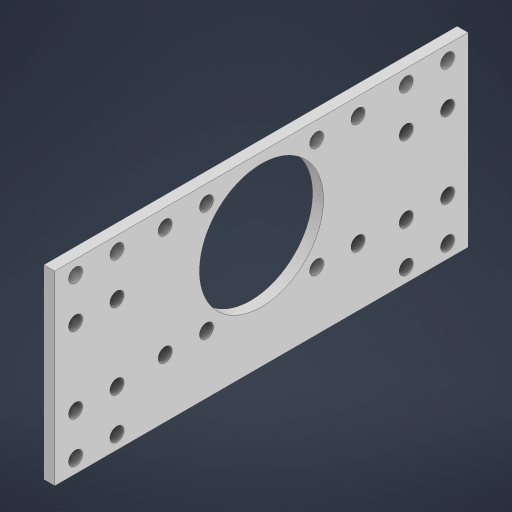
# Autodesk Inventor part: TurretMotorCase_SidePlate
Saved by Autodesk Inventor 2024 (Build 280153000, 153)
## iProperties
Created: 2023-10-26
Part Number: TurretMotorCase_SidePlate
Material: Generic
Document SubType Name: Modeling
Designer: avsar
Density: 1 g/cm^3
Appearance: Default
Author: avsar
Autodesk Inventor part; units mm, degrees
ref_plane "YZ Plane" through (0, 0, 0) normal (1, 0, 0) x (0, 1, 0)
ref_plane "XZ Plane" through (0, 0, 0) normal (0, 1, 0) x (-1, 0, 0)
ref_plane "XY Plane" through (0, 0, 0) normal (0, 0, 1) x (1, 0, 0)
sketch "Sketch1" plane through (0, 0, 0) normal (1, 0, 0) x (0, 1, 0)
  line L0 (-27, 60) -> (27, 60)
  line L1 (27, 60) -> (27, -60)
  line L2 (27, -60) -> (-27, -60)
  line L3 (-27, -60) -> (-27, 60)
  line L4 (-27, 60) -> (27, -60) construction
  line L5 (27, 60) -> (-27, -60) construction
  point P0 (0, 0)
  dimension "d0" = 54
  dimension "d1" = 120
  constraints: 12 end point, 2 midpoint, 2 parallel, 1 horizontal, 1 perpendicular
  measures "d0" distance of L1.end L2.end
  measures "d1" distance of L0.end L1.end
extrude "Extrusion1" add sketch "Sketch1" along normal mid plane 3.175
sketch "Sketch2" plane through (1.5875, 0, 0) normal (1, 0, 0) x (0, 0, -1)
  circle A0 centre (-48, -17) radius 2.5 construction
  line L0 (-60, -27) -> (60, -27) construction
  circle A1 centre (-54, -23) radius 2
  circle A2 centre (-42, -23) radius 2
  circle A3 centre (-42, -11) radius 2
  circle A4 centre (-54, -11) radius 2
  line L1 (0, 27) -> (0, -27) construction
  line L2 (60, 27) -> (-60, 27) construction
  line L3 (-60, 27) -> (-60, -27) construction
  line L4 (60, -27) -> (60, 27) construction
  line L5 (-60, 0) -> (60, 0) construction
  circle A5 centre (54, -23) radius 2
  circle A6 centre (42, -23) radius 2
  circle A7 centre (42, -11) radius 2
  circle A8 centre (54, -11) radius 2
  circle A9 centre (-54, 23) radius 2
  circle A10 centre (-42, 23) radius 2
  circle A11 centre (-42, 11) radius 2
  circle A12 centre (-54, 11) radius 2
  circle A13 centre (54, 11) radius 2
  circle A14 centre (42, 11) radius 2
  circle A15 centre (54, 23) radius 2
  circle A16 centre (42, 23) radius 2
  point P0 (0, 0)
  dimension "d4" = 5
  dimension "d5" = 48
  dimension "d6" = 10
  dimension "d7" = 4
  dimension "d8" = 6
  dimension "d9" = 6
  dimension "d12" = 360
  constraints: 17 centre point, 12 symmetric about line, 4 end point, 4 midpoint, 21 other
  measures "d4" diameter of A0
  measures "d5" horizontal distance of point (0, 0) A0.centre
  measures "d6" distance from line of L0 A0.centre
  measures "d7" diameter of A1
  measures "d8" horizontal distance of A0.centre A1.centre
  measures "d9" horizontal distance of A0.centre A1.centre
extrude "Extrusion2" cut sketch "Sketch2" against normal through all
sketch "Sketch4" plane through (1.5875, 0, 0) normal (1, 0, 0) x (0, 0, -1)
  circle A0 centre (0, 6) radius 18
  circle A1 centre (-28, 22) radius 2
  line L0 (0, 24) -> (0, -12) construction
  line L1 (60, 27) -> (-60, 27) construction
  line L2 (-18, 6) -> (18, 6) construction
  circle A2 centre (-16, 22) radius 2
  circle A3 centre (28, 22) radius 2
  circle A4 centre (-28, -10) radius 2
  circle A5 centre (28, -10) radius 2
  circle A6 centre (-16, -10) radius 2
  circle A7 centre (16, -10) radius 2
  circle A8 centre (16, 22) radius 2
  point P0 (0, 0)
  dimension "d30" = 36
  dimension "d31" = 6
  dimension "d32" = 4
  dimension "d33" = 28
  dimension "d34" = 16
  dimension "d35" = 4
  dimension "d36" = 16
  dimension "d37" = 16
  dimension "d40" = 360
  constraints: 9 centre point, 4 end point, 4 point on circle, 3 symmetric about line, 2 midpoint, 1 coincident, 1 horizontal, 1 perpendicular, 1 vertical alignment, 12 other
  measures "d30" diameter of A0
  measures "d31" distance of point (0, 0) A0.centre
  measures "d32" diameter of A1
  measures "d33" horizontal distance of A1.centre A0.centre
  measures "d34" vertical distance of A0.centre A1.centre
  measures "d35" diameter of A2
  measures "d36" horizontal distance of A0.centre A2.centre
  measures "d37" horizontal distance of A0.centre A2.centre
extrude "Extrusion4" cut sketch "Sketch4" against normal through all
body "Solid1"
